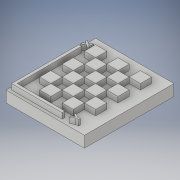
# Autodesk Inventor part: 3D_Grid
Saved by Autodesk Inventor 2019 (Build 230136000, 136)
## iProperties
Created: 2019-06-17
Part Number: 3D_Grid
Material: Generic
Document SubType Name: Modeling
Designer: David
Density: 1 g/cm^3
Appearance: Default
Author: David
Autodesk Inventor part; units mm, degrees
ref_plane "YZ Plane" through (0, 0, 0) normal (1, 0, 0) x (0, 1, 0)
ref_plane "XZ Plane" through (0, 0, 0) normal (0, 1, 0) x (-1, 0, 0)
ref_plane "XY Plane" through (0, 0, 0) normal (0, 0, 1) x (1, 0, 0)
sketch "Sketch1" plane through (0, 0, 0) normal (0, 1, 0) x (-1, 0, 0)
  line L0 (70, 80) -> (-70, 80)
  line L1 (-70, 80) -> (-70, -80)
  line L2 (-70, -80) -> (70, -80)
  line L3 (70, -80) -> (70, 80)
  point P0 (0, 0)
  dimension "d0" = 140
  dimension "d1" = 160
  dimension "d4" = 70
  dimension "d5" = 80
  constraints: 8 end point, 2 parallel, 1 horizontal, 1 perpendicular
  measures "d0" distance between parallel lines of L1 L3
  measures "d1" distance between parallel lines of L2 L0
  measures "d4" distance from line of point (0, 0) L1
  measures "d5" distance from line of point (0, 0) L2
extrude "Extrusion1" add sketch "Sketch1" along normal blind 20
sketch "Sketch2" plane through (0, 20, 0) normal (0, 1, 0) x (1, 0, 0)
  line L0 (50, 60) -> (-50, 60)
  line L1 (-50, 60) -> (-50, -60)
  line L2 (-50, -60) -> (50, -60)
  line L3 (50, -60) -> (50, 60)
  line L4 (50, 60) -> (-50, -60) construction
  line L5 (-50, 60) -> (50, -60) construction
  point P0 (0, 0)
  dimension "d8" = 100
  dimension "d9" = 120
  constraints: 12 end point, 2 midpoint, 2 parallel, 1 horizontal, 1 perpendicular
  measures "d8" distance of L1.end L2.end
  measures "d9" distance of L0.end L1.end
extrude "Extrusion2" add sketch "Sketch2" along normal blind 10
sketch "Sketch3" plane through (0, 30, 0) normal (0, 1, 0) x (1, 0, 0)
  line L0 (-50, 60) -> (-50, -60) projected
  line L1 (-50, -60) -> (-30, -60)
  line L2 (-30, -60) -> (-30, -40)
  line L3 (-30, -40) -> (-50, -40)
  line L4 (-50, -40) -> (-50, -60)
  line L5 (-10, -60) -> (10, -60)
  line L6 (10, -60) -> (10, -40)
  line L7 (10, -40) -> (-10, -40)
  line L8 (-10, -40) -> (-10, -60)
  line L9 (10, -40) -> (30, -40)
  line L10 (30, -40) -> (30, -20)
  line L11 (30, -20) -> (10, -20)
  line L12 (10, -20) -> (10, -40)
  line L13 (-30, -40) -> (-10, -40)
  line L14 (-10, -40) -> (-10, -20)
  line L15 (-10, -20) -> (-30, -20)
  line L16 (-30, -20) -> (-30, -40)
  line L17 (-50, -60) -> (50, -60) projected
  line L18 (-53.5785, -189.3047) -> (-33.5785, -189.3047)
  line L19 (-33.5785, -189.3047) -> (-33.5785, -169.3047)
  line L20 (-33.5785, -169.3047) -> (-53.5785, -169.3047)
  line L21 (-53.5785, -169.3047) -> (-53.5785, -189.3047)
  line L22 (-50, -20) -> (-30, -20)
  line L23 (-30, -20) -> (-30, 0)
  line L24 (-30, 0) -> (-50, 0)
  line L25 (-50, 0) -> (-50, -20)
  line L26 (-10, -20) -> (10, -20)
  line L27 (10, -20) -> (10, 0)
  line L28 (10, 0) -> (-10, 0)
  line L29 (-10, 0) -> (-10, -20)
  line L30 (10, 40) -> (30, 40)
  line L31 (30, 40) -> (30, 60)
  line L32 (30, 60) -> (10, 60)
  line L33 (10, 60) -> (10, 40)
  line L34 (-10, 20) -> (-30, 20)
  line L35 (-30, 0) -> (-10, 0)
  line L36 (-30, 20) -> (-30, 0)
  line L37 (-10, 0) -> (-10, 20)
  line L38 (10, 40) -> (-10, 40)
  line L39 (-10, 20) -> (10, 20)
  line L40 (-10, 40) -> (-10, 20)
  line L41 (10, 20) -> (10, 40)
  line L42 (30, 20) -> (10, 20)
  line L43 (10, 0) -> (30, 0)
  line L44 (10, 20) -> (10, 0)
  line L45 (30, 0) -> (30, 20)
  line L46 (-10, 60) -> (-30, 60)
  line L47 (-30, 40) -> (-10, 40)
  line L48 (-30, 60) -> (-30, 40)
  line L49 (-10, 40) -> (-10, 60)
  line L50 (-30, 40) -> (-50, 40)
  line L51 (-50, 20) -> (-30, 20)
  line L52 (-50, 40) -> (-50, 20)
  line L53 (-30, 20) -> (-30, 40)
  line L54 (30, 20) -> (50, 20)
  line L55 (50, 20) -> (50, 40)
  line L56 (50, 40) -> (30, 40)
  line L57 (30, 40) -> (30, 20)
  line L58 (30, -20) -> (50, -20)
  line L59 (50, -20) -> (50, 0)
  line L60 (50, 0) -> (30, 0)
  line L61 (30, 0) -> (30, -20)
  line L62 (30, -60) -> (50, -60)
  line L63 (50, -60) -> (50, -40)
  line L64 (50, -40) -> (30, -40)
  line L65 (30, -40) -> (30, -60)
  dimension "d12" = 20
  dimension "d13" = 20
  dimension "d14" = 20
  dimension "d15" = 20
  dimension "d17" = 20
  dimension "d18" = 20
  dimension "d19" = 20
  dimension "d21" = 20
  dimension "d22" = 20
  dimension "d25" = 20
  dimension "d26" = 20
  dimension "d27" = 20
  dimension "d28" = 20
  dimension "d30" = 20
  dimension "d31" = 20
  dimension "d33" = 20
  dimension "d34" = 20
  dimension "d36" = 20
  dimension "d37" = 20
  dimension "d39" = 20
  dimension "d40" = 20
  dimension "d42" = 20
  dimension "d43" = 20
  dimension "d45" = 20
  dimension "d46" = 20
  dimension "d48" = 20
  dimension "d49" = 20
  dimension "d77" = 20
  dimension "d78" = 20
  dimension "d80" = 20
  dimension "d81" = 20
  dimension "d83" = 20
  dimension "d84" = 20
  constraints: 128 end point, 32 parallel, 16 horizontal, 15 perpendicular, 1 coincident
  measures "d12" distance of L2.end L3.end
  measures "d13" distance of L1.end L2.end
  measures "d14" distance of L6.end L7.end
  measures "d15" distance of L6.end L5.end
  measures "d17" distance of L7.end L2.end
  measures "d18" distance of L10.end L11.end
  measures "d19" distance of L9.end L10.end
  measures "d21" distance of L14.end L16.start
  measures "d22" distance of L14.start L14.end
  measures "d25" distance of L18.end L19.end
  measures "d26" distance of L19.end L20.end
  measures "d27" distance of L16.start L24.start
  measures "d28" distance of L24.start L24.end
  measures "d30" distance of L26.end L28.start
  measures "d31" distance of L28.start L28.end
  measures "d33" distance of L30.end L32.start
  measures "d34" distance of L32.start L32.end
  measures "d36" distance of L37.start L34.start
  measures "d37" distance of L34.start L34.end
  measures "d39" distance of L41.start L30.start
  measures "d40" distance of L30.start L38.end
  measures "d42" distance of L45.start L42.start
  measures "d43" distance of L42.start L41.start
  measures "d45" distance of L38.end L46.start
  measures "d46" distance of L46.start L46.end
  measures "d48" distance of L34.end L50.start
  measures "d49" distance of L50.start L50.end
  measures "d77" distance of L55.start L56.start
  measures "d78" distance of L30.end L56.start
  measures "d80" distance of L59.start L60.start
  measures "d81" distance of L45.start L60.start
  measures "d83" distance of L63.start L64.start
  measures "d84" distance of L9.end L64.start
extrude "Extrusion5" cut sketch "Sketch3" against normal blind 10 contours L50 L53 L51 L0 | L48 L46 L49 L47 | L24 L23 L22 L0 | L34 L37 L35 L36 | L38 L41 L39 L40 | L33 L32 L31 L30 | L3 L2 L1 L0 | L15 L14 L13 L16 | L28 L27 L26 L29 | L42 L45 L43 L44 | L56 L55 L54 L57 | L7 L6 L5 L8 | L11 L10 L9 L12 | L60 L59 L58 L61 | L64 L63 L17 L65
sketch "Sketch4" plane through (0, 20, 0) normal (0, 1, 0) x (1, 0, 0)
  line L0 (-65, -75) -> (-65, 45)
  line L1 (-65, 45) -> (-60, 45)
  line L2 (-60, 45) -> (-60, -70)
  line L3 (-60, -70) -> (25, -70)
  line L4 (25, -70) -> (25, -75)
  line L5 (25, -75) -> (-65, -75)
  line L6 (-70, -80) -> (70, -80) projected
  line L7 (-70, 80) -> (-70, -80) projected
  line L8 (-52.7495, 59.3949) -> (-52.7495, 49.2445) construction
  line L9 (-52.7495, 49.2445) -> (-65, 49.2445) construction
  line L10 (-65, 49.2445) -> (-65, 59.3949) construction
  line L11 (-65, 59.3949) -> (-52.7495, 59.3949) construction
  line L12 (38.6741, -75) -> (38.6741, -63.6245) construction
  line L13 (38.6741, -63.6245) -> (40.6911, -63.6245) construction
  line L14 (40.6911, -63.6245) -> (40.6911, -75) construction
  line L15 (40.6911, -75) -> (38.6741, -75) construction
  line L16 (-64.7495, 47.9979) -> (-64.7495, 51.4792)
  line L17 (-64.7495, 51.4792) -> (-60.9278, 53.7936)
  line L18 (-60.9278, 53.7936) -> (-64.7495, 56.1567)
  line L19 (-64.7495, 56.1567) -> (-64.7495, 59.4922)
  line L20 (-64.7495, 59.4922) -> (-58.7106, 55.5927)
  line L21 (-58.7106, 55.5927) -> (-52.7495, 59.3366)
  line L22 (-52.7495, 59.3366) -> (-52.7495, 55.8552)
  line L23 (-52.7495, 55.8552) -> (-56.3767, 53.6867)
  line L24 (-56.3767, 53.6867) -> (-52.7495, 51.4598)
  line L25 (-52.7495, 51.4598) -> (-52.7495, 48.1243)
  line L26 (-52.7495, 48.1243) -> (-58.5842, 51.8877)
  line L27 (-58.5842, 51.8877) -> (-64.7495, 47.9979)
  line L28 (38.6741, -63.778) -> (45.666, -67.9206)
  line L29 (45.666, -67.9206) -> (50.6741, -67.9206)
  line L30 (50.6741, -67.9206) -> (50.6741, -70.9352)
  line L31 (50.6741, -70.9352) -> (45.8119, -70.9352)
  line L32 (45.8119, -70.9352) -> (38.6741, -75.1459)
  line L33 (38.6741, -75.1459) -> (38.6741, -71.7131)
  line L34 (38.6741, -71.7131) -> (42.9529, -69.3695)
  line L35 (42.9529, -69.3695) -> (38.6741, -67.1037)
  line L36 (38.6741, -67.1037) -> (38.6741, -63.778)
  point P0 (0, 0)
  point P1 (-62.5, 45)
  point P2 (-58.8748, 54.3197)
  point P3 (25, -72.5)
  point P4 (34.4783, -69.3123)
  point P5 (-58.8748, 54.3197)
  point P6 (34.4783, -69.3123)
  dimension "d53" = 5
  dimension "d54" = 5
  dimension "d55" = 5
  dimension "d56" = 5
  dimension "d57" = 120
  dimension "d58" = 90
  dimension "d59" = 10
  dimension "d60" = 10
  dimension "d62" = 10.1504
  dimension "d63" = 12.2505
  dimension "d64" = 5.0752
  dimension "d65" = 6.1252
  dimension "d68" = 5.6877
  dimension "d70" = 6.2127
  dimension "d71" = 5.6877
  dimension "d73" = 5
  dimension "d74" = 5
  constraints: 12 end point, 5 perpendicular, 2 coincident, 2 midpoint, 1 vertical, 4 other
  measures "d53" distance between parallel lines of L2 L0
  measures "d54" distance between parallel lines of L5 L3
  measures "d55" distance between parallel lines of L6 L5
  measures "d56" distance between parallel lines of L7 L0
  measures "d57" distance of L0.start L0.end
  measures "d58" distance of L4.end L0.start
  measures "d59" distance of point (-62.5, 45) point (-58.875, 54.32)
  measures "d60" distance of point (34.478, -69.312) point (25, -72.5)
  measures "d62" distance of L8.start L8.end
  measures "d63" distance of L8.end L9.end
  measures "d64" distance from line of L9 point (-58.875, 54.32)
  measures "d65" distance from line of L8 point (-58.875, 54.32)
  measures "d68" distance from line of L15 point (34.478, -69.312)
  measures "d70" distance from line of L14 point (34.478, -69.312)
  measures "d71" distance from line of L13 point (34.478, -69.312)
  measures "d73" distance between parallel lines of L6 L15
  measures "d74" distance between parallel lines of L10 L7
extrude "Extrusion4" add sketch "Sketch4" along normal blind 10
equation "\"d4\" = 0.5 * d0"
equation "\"d5\" = 0.5 * d1"
equation "\"d12\" = cell"
equation "\"d13\" = cell"
equation "\"d14\" = d16"
equation "\"d15\" = d16"
equation "\"d17\" = cell"
equation "\"d18\" = d20"
equation "\"d19\" = d20"
equation "\"d21\" = d23"
equation "\"d22\" = d23"
equation "\"d25\" = cell"
equation "\"d26\" = cell"
equation "\"d27\" = d29"
equation "\"d28\" = d29"
equation "\"d30\" = d32"
equation "\"d31\" = d32"
equation "\"d33\" = d35"
equation "\"d34\" = d35"
equation "\"d36\" = d38"
equation "\"d37\" = d38"
equation "\"d39\" = d41"
equation "\"d40\" = d41"
equation "\"d42\" = d44"
equation "\"d43\" = d44"
equation "\"d45\" = d47"
equation "\"d46\" = d47"
equation "\"d48\" = d50"
equation "\"d49\" = d50"
equation "\"cell\" = 20"
equation "\"d16\" = 20"
equation "\"d20\" = 20"
equation "\"d23\" = 20"
equation "\"d29\" = 20"
equation "\"d32\" = 20"
equation "\"d35\" = 20"
equation "\"d38\" = 20"
equation "\"d41\" = 20"
equation "\"d44\" = 20"
equation "\"d47\" = 20"
equation "\"d50\" = 20"
body "Solid1"
